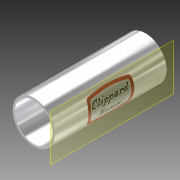
# Autodesk Inventor part: Accumulator Tank 1764
Saved by Autodesk Inventor 2011 (Build 150239000, 239)
## iProperties
Created: 2010-01-18
Part Number: Accumulator Tank 1764
Document SubType Name: Modeling
Designer: cmcfadden
Density: 1 g/cm^3
Author: cmcfadden
Autodesk Inventor part; units mm, degrees
ref_plane "XZ Plane" through (0, 0, 0) normal (0, 1, 0) x (-1, 0, 0)
ref_plane "XY Plane" through (0, 0, 0) normal (0, 0, 1) x (1, 0, 0)
sketch "Sketch1" plane through (0, 0, 0) normal (0, 0, 1) x (1, 0, 0)
  circle A0 centre (10.4262, -13.0137) radius 26.416
  point P0 (0, 0)
  dimension "d0" = 52.832
  constraints: 1 centre point
  measures "d0" diameter of A0
extrude "Extrusion1" add sketch "Sketch1" along normal blind 139.7508
ref_plane "Work Plane1" through (38.1, 0, 0) normal (1, 0, 0) x (0, 1, 0)
sketch "Sketch2" plane through (38.1, 0, 0) normal (1, 0, 0) x (0, 1, 0)
  point P0 (0, 0)
sketch "Sketch3" plane through (10.4262, -13.0137, 139.7508) normal (0, 0, 1) x (1, 0, 0)
  circle A0 centre (0, 0) radius 26.416 projected
  circle A1 centre (0, 0) radius 23.6474
  point P0 (-10.4262, 13.0137)
  dimension "d14" = 47.2948
  constraints: 1 centre point, 1 coincident
  measures "d14" diameter of A1
extrude "Extrusion2" cut sketch "Sketch3" against normal through all contours A1
sketch "Sketch4" plane through (38.1, 0, 0) normal (1, 0, 0) x (0, 1, 0)
  line L0 (-39.4297, 139.7508) -> (13.4023, 139.7508) projected
  line L1 (-39.4297, 0) -> (13.4023, 0) projected
  line L2 (13.4023, 0) -> (13.4023, 139.7508) projected
  line L3 (-39.4297, 0) -> (-39.4297, 139.7508) projected
  line L4 (6.3845, 98.8211) -> (6.3845, 39.2899) construction
  line L5 (6.3845, 39.2899) -> (-32.2447, 39.2899) construction
  line L6 (-32.2447, 39.2899) -> (-32.2447, 98.8211) construction
  line L7 (-32.2447, 98.8211) -> (6.3845, 98.8211) construction
  point P0 (0, 0)
  constraints: 2 other
decal "Decal1"
body "Solid1"
